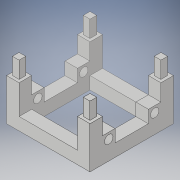
# Autodesk Inventor part: 000.113 - Верх центрального сегмента
Saved by Autodesk Inventor 2019 (Build 230136000, 136)
## iProperties
Created: 2020-06-07
Part Number: 000.113 - Верх центрального сегмента
Material: Типовые
Document SubType Name: Modeling
Designer: Петров Иван
Density: 1 g/cm^3
Appearance: По умолчанию
Author: Петров Иван
Autodesk Inventor part; units mm, degrees
ref_plane "YZ Plane" through (0, 0, 0) normal (1, 0, 0) x (0, 1, 0)
ref_plane "XZ Plane" through (0, 0, 0) normal (0, 1, 0) x (-1, 0, 0)
ref_plane "XY Plane" through (0, 0, 0) normal (0, 0, 1) x (1, 0, 0)
sketch "Эскиз1" plane through (0, 0, 0) normal (0, 1, 0) x (-1, 0, 0)
  line L0 (-50, 50) -> (50, 50)
  line L1 (50, 50) -> (50, -50)
  line L2 (50, -50) -> (-50, -50)
  line L3 (-50, -50) -> (-50, 50)
  line L4 (-50, 50) -> (50, -50) construction
  line L5 (50, 50) -> (-50, -50) construction
  line L6 (-35, 35) -> (35, 35)
  line L7 (35, 35) -> (35, -35)
  line L8 (35, -35) -> (-35, -35)
  line L9 (-35, -35) -> (-35, 35)
  line L10 (-35, 35) -> (35, -35) construction
  line L11 (35, 35) -> (-35, -35) construction
  point P0 (0, 0)
  dimension "d0" = 100
  dimension "d1" = 100
  dimension "d2" = 15
  dimension "d3" = 15
  constraints: 24 end point, 4 midpoint, 4 parallel, 2 horizontal, 2 perpendicular
  measures "d0" distance of L1.end L2.end
  measures "d1" distance of L0.end L1.end
  measures "d2" distance between parallel lines of L1 L7
  measures "d3" distance between parallel lines of L2 L8
extrude "Выдавливание1" add sketch "Эскиз1" along normal blind 50
sketch "Эскиз3" plane through (0, 50, 0) normal (0, 1, 0) x (1, 0, 0)
  line L0 (-35, 35) -> (-35, -35) projected
  line L1 (-35, 0) -> (-50, 0)
  line L2 (-50, -50) -> (-50, 50) projected
  line L3 (35, -35) -> (35, 35) projected
  line L4 (35, 0) -> (50, 0)
  line L5 (50, 50) -> (50, -50) projected
  line L6 (-35, -20) -> (-50, -20)
  line L7 (-50, -20) -> (-50, 20)
  line L8 (-50, 20) -> (-35, 20)
  line L9 (-35, 20) -> (-35, -20)
  line L10 (-35, -20) -> (-50, 20) construction
  line L11 (-50, -20) -> (-35, 20) construction
  line L12 (50, -20) -> (35, -20)
  line L13 (35, -20) -> (35, 20)
  line L14 (35, 20) -> (50, 20)
  line L15 (50, 20) -> (50, -20)
  line L16 (50, -20) -> (35, 20) construction
  line L17 (35, -20) -> (50, 20) construction
  line L18 (-35, -35) -> (35, -35) projected
  line L19 (0, -35) -> (0, -50)
  line L20 (50, -50) -> (-50, -50) projected
  line L21 (35, 35) -> (-35, 35) projected
  line L22 (0, 35) -> (0, 50)
  line L23 (-50, 50) -> (50, 50) projected
  line L24 (35, -50) -> (-35, -50)
  line L25 (-35, -50) -> (-35, -35)
  line L26 (-35, -35) -> (35, -35)
  line L27 (35, -35) -> (35, -50)
  line L28 (35, -50) -> (-35, -35) construction
  line L29 (-35, -50) -> (35, -35) construction
  line L30 (35, 50) -> (-35, 50)
  line L31 (-35, 50) -> (-35, 35)
  line L32 (-35, 35) -> (35, 35)
  line L33 (35, 35) -> (35, 50)
  line L34 (35, 50) -> (-35, 35) construction
  line L35 (-35, 50) -> (35, 35) construction
  point P0 (0, 0)
  point P1 (-42.5, 0)
  point P2 (42.5, 0)
  point P3 (0, -42.5)
  point P4 (0, 42.5)
  dimension "d14" = 40
  dimension "d15" = 40
  constraints: 56 end point, 20 midpoint, 8 parallel, 4 horizontal, 4 perpendicular, 2 point on line
  measures "d14" distance of L6.end L7.end
  measures "d15" distance of L12.end L13.end
extrude "Выдавливание2" cut sketch "Эскиз3" against normal blind 35 contours L31 L23 L22 L21 | L0 L1 L2 L8 | L22 L23 L33 L21 | L0 L6 L2 L1 | L14 L5 L4 L3 | L18 L19 L20 L25 | L4 L5 L12 L3 | L18 L27 L20 L19
sketch "Эскиз4" plane through (-35, 0, 35) normal (1, 0, 0) x (0, 0, -1)
  line L0 (15, 15) -> (15, 50) projected
  line L1 (15, 50) -> (0, 50)
  line L2 (0, 50) -> (0, 30)
  line L3 (0, 30) -> (15, 30)
  line L4 (15, 30) -> (15, 50)
  line L5 (85, 50) -> (55, 50) projected
  line L6 (55, 50) -> (70, 50)
  line L7 (70, 50) -> (70, 30)
  line L8 (70, 30) -> (55, 30)
  line L9 (55, 30) -> (55, 50)
  point P0 (35, 0)
  dimension "d18" = 15
  dimension "d19" = 20
  dimension "d20" = 15
  dimension "d21" = 20
  constraints: 16 end point, 4 parallel, 2 horizontal, 2 perpendicular
  measures "d18" distance of L3.end L2.end
  measures "d19" distance of L2.end L1.end
  measures "d20" distance of L7.end L8.end
  measures "d21" distance of L6.end L7.end
extrude "Выдавливание3" cut sketch "Эскиз4" along normal blind 90.5 and the other way blind 45.25
sketch "Эскиз5" plane through (50, 0, 50) normal (1, 0, 0) x (0, 0, -1)
  circle A0 centre (22.5, 22.5) radius 5.1
  circle A1 centre (77.5, 22.5) radius 5.1
  line L0 (85, 30) -> (70, 30) projected
  line L1 (70, 30) -> (70, 15) projected
  line L2 (30, 15) -> (30, 30) projected
  line L3 (30, 30) -> (15, 30) projected
  point P0 (50, 0)
  dimension "d26" = 10.2
  dimension "d27" = 10.2
  dimension "d28" = 7.5
  dimension "d29" = 7.5
  dimension "d30" = 7.5
  dimension "d31" = 7.5
  constraints: 2 centre point
  measures "d26" diameter of A0
  measures "d27" diameter of A1
  measures "d28" distance from line of L0 A1.centre
  measures "d29" distance from line of L1 A1.centre
  measures "d30" distance from line of L2 A0.centre
  measures "d31" distance from line of L3 A0.centre
extrude "Выдавливание4" cut sketch "Эскиз5" against normal blind 156
sketch "Эскиз6" plane through (0, 50, 0) normal (0, 1, 0) x (1, 0, 0)
  line L0 (-35, 35) -> (-50, 35) projected
  line L1 (-50, 50) -> (50, 50) projected
  line L2 (-38.5, 46.5) -> (-46.5, 46.5)
  line L3 (-46.5, 46.5) -> (-46.5, 38.5)
  line L4 (-46.5, 38.5) -> (-38.5, 38.5)
  line L5 (-38.5, 38.5) -> (-38.5, 46.5)
  line L6 (-38.5, 46.5) -> (-46.5, 38.5) construction
  line L7 (-46.5, 46.5) -> (-38.5, 38.5) construction
  line L8 (-50, 50) -> (-50, 35) projected
  point P0 (0, 0)
  point P1 (-42.5, 42.5)
  dimension "d34" = 8
  dimension "d35" = 8
  dimension "d41" = 7.5
  dimension "d42" = 7.5
  constraints: 12 end point, 2 midpoint, 2 parallel, 1 horizontal, 1 perpendicular
  measures "d34" distance of L4.end L3.end
  measures "d35" distance of L3.end L2.end
  measures "d41" distance from line of L1 point (-42.5, 42.5)
  measures "d42" distance from line of L8 point (-42.5, 42.5)
extrude "Выдавливание5" add sketch "Эскиз6" along normal blind 20
mirror "Mirror1" about plane through (0, 0, 0) normal (1, 0, 0) of "Выдавливание5"
mirror "Mirror2" about plane through (0, 0, 0) normal (0, 0, 1) of "Выдавливание5", "Mirror1"
